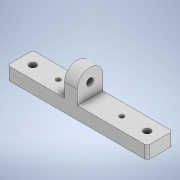
# Autodesk Inventor part: リアルセンスマウント1
Saved by Autodesk Inventor 2020 (Build 240168000, 168)
## iProperties
Created: 2019-10-27
Part Number: リアルセンスマウント1
Material: 一般
Document SubType Name: Modeling
Designer: highs
Density: 1 g/cm^3
Appearance: 既定
Author: highs
## iProperties of the stored document _3D プリント.ipt
Created: 2019-10-28
Part Number: _3D プリント
Material: 一般
Document SubType Name: Modeling
Designer: highs
Density: 1 g/cm^3
Appearance: 既定
Author: highs
Autodesk Inventor part; units mm, degrees
ref_plane "YZ Plane" through (0, 0, 0) normal (1, 0, 0) x (0, 1, 0)
ref_plane "XZ Plane" through (0, 0, 0) normal (0, 1, 0) x (-1, 0, 0)
ref_plane "XY Plane" through (0, 0, 0) normal (0, 0, 1) x (1, 0, 0)
sketch "スケッチ1" plane through (0, 0, 0) normal (0, 0, 1) x (1, 0, 0)
  line L0 (0, 0) -> (110, 0)
  line L1 (110, 0) -> (110, 10)
  line L2 (110, 10) -> (55, 10)
  line L3 (55, 10) -> (55, 31)
  line L4 (55, 31) -> (45, 31)
  line L5 (45, 31) -> (45, 10)
  line L6 (45, 10) -> (0, 10)
  line L7 (0, 10) -> (0, 0)
  dimension "d0" = 110
  dimension "d1" = 10
  dimension "d2" = 21
  dimension "d3" = 10
  dimension "d4" = 45
  constraints: 16 end point, 6 perpendicular, 2 point on line, 1 horizontal
  measures "d0" distance of L0.start L0.end
  measures "d1" distance of L6.end L0.start
  measures "d2" distance of L4.end L5.end
  measures "d3" distance of L3.end L4.end
  measures "d4" distance between parallel lines of L7 L5
extrude "押し出し1" add sketch "スケッチ1" along normal blind 20
sketch "スケッチ2" plane through (0, 0, 0) normal (0, -1, 0) x (1, 0, 0)
  line L0 (110, 0) -> (110, 20) construction
  line L1 (110, 10) -> (0, 10) construction
  line L2 (0, 0) -> (0, 20) construction
  circle A0 centre (100, 10) radius 2.75
  circle A1 centre (10, 10) radius 2.75
  line L3 (0, 0) -> (110, 0) construction
  line L4 (55, 0) -> (55, 20) construction
  line L5 (0, 20) -> (110, 20) construction
  circle A2 centre (80, 10) radius 1.75
  circle A3 centre (30, 10) radius 1.75
  dimension "d7" = 5.5
  dimension "d8" = 10
  dimension "d9" = 10
  dimension "d17" = 3.5
  dimension "d18" = 50
  constraints: 4 centre point, 4 end point, 4 midpoint, 3 point on line, 1 equal radius, 1 symmetric about line, 1 other
  measures "d7" diameter of A0
  measures "d8" distance from line of L0 A0.centre
  measures "d9" distance from line of L2 A1.centre
  measures "d17" diameter of A2
  measures "d18" distance of A3.centre A2.centre
extrude "押し出し2" cut sketch "スケッチ2" against normal through all
sketch "スケッチ3" plane through (45, 10, 0) normal (-1, 0, 0) x (0, 0, 1)
  line L0 (0, 21) -> (20, 21) construction
  line L1 (10, 21) -> (10, 0) construction
  line L2 (0, 0) -> (20, 0) construction
  circle A0 centre (10, 11) radius 2.75
  point P0 (0, -10)
  dimension "d12" = 10
  dimension "d13" = 5.5
  constraints: 2 end point, 2 midpoint, 1 centre point, 1 point on line
  measures "d12" distance from line of L0 A0.centre
  measures "d13" diameter of A0
extrude "押し出し3" cut sketch "スケッチ3" against normal through all
fillet "フィレット1" radius 10 2 edges at (50, 31, 0) (50, 31, 20)
fillet "フィレット2" radius 2 4 edges at (110, 5, 20) (110, 5, 0) (0, 5, 0) (0, 5, 20)
